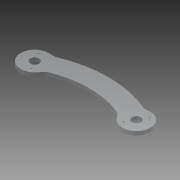
# Autodesk Inventor part: Femur
Saved by Autodesk Inventor 2015 (Build 190159000, 159)
## iProperties
Created: 2015-10-11
Part Number: Femur
Material: Generic
Document SubType Name: Modeling
Designer: styku
Density: 1 g/cm^3
Appearance: Clear - Blue
Mass: 4.92784 g
Surface Area: 41.7146 cm^2
Volume: 4.92784 cm^3
Author: styku
Autodesk Inventor part; units mm, degrees
ref_plane "YZ Plane" through (0, 0, 0) normal (1, 0, 0) x (0, 1, 0)
ref_plane "XZ Plane" through (0, 0, 0) normal (0, 1, 0) x (-1, 0, 0)
ref_plane "XY Plane" through (0, 0, 0) normal (0, 0, 1) x (1, 0, 0)
sketch "Sketch1" plane through (0, 0, 0) normal (0, 0, 1) x (1, 0, 0)
  line L0 (0, 107) -> (0, -103) construction
  line L1 (-117, 0) -> (116, 0) construction
  arc A0 (-38.3571, 10.8766) -> (-30.6918, -5.8614) centre (-40, 0) ccw
  arc A1 (30.6918, -5.8614) -> (38.3571, 10.8766) centre (40, 0) ccw
  arc A2 (40, 0) -> (-40, 0) centre (0, -69.282) ccw construction
  line L2 (-40, 13) -> (-40, -15) construction
  line L3 (40, 13) -> (40, -15) construction
  arc A3 (25.8036, -1.8505) -> (-25.8036, -1.8505) centre (0, -69.282) ccw
  arc A4 (33.0749, 11.5099) -> (-33.0749, 11.5099) centre (0, -69.282) ccw
  arc A5 (-38.3571, 10.8766) -> (-33.0749, 11.5099) centre (-36.8635, 20.7645) ccw
  arc A6 (-25.8036, -1.8505) -> (-30.6918, -5.8614) centre (-22.2297, -11.19) ccw
  arc A7 (33.0749, 11.5099) -> (38.3571, 10.8766) centre (36.8635, 20.7645) ccw
  arc A8 (30.6918, -5.8614) -> (25.8036, -1.8505) centre (22.2297, -11.19) ccw
  line L4 (-39.7655, 0.1354) -> (-60.5453, -11.8618) construction
  line L5 (-46.3958, 11.0778) -> (-33.6042, -11.0778) construction
  circle A9 centre (-43.75, 6.4952) radius 0.5
  circle A10 centre (-36.25, -6.4952) radius 0.5
  circle A11 centre (43.75, 6.4952) radius 0.5
  circle A12 centre (36.25, -6.4952) radius 0.5
  circle A13 centre (-40, 0) radius 3.5
  circle A14 centre (40, 0) radius 3.5
  point P0 (0, 0)
  dimension "d0" = 22
  dimension "d1" = 40
  dimension "d2" = 80
  dimension "d6" = 10
  dimension "d7" = 72.2
  dimension "d8" = 87.3
  dimension "d9" = 1
  dimension "d10" = 7.5
  dimension "d11" = 7
  constraints: 18 point on circle, 15 centre point, 12 end point, 9 tangent, 7 symmetric about line, 4 point on line, 3 equal radius, 2 concentric, 2 horizontal, 2 perpendicular, 2 vertical, 1 coincident, 1 midpoint, 5 other
  measures "d0" diameter of A0
  measures "d1" distance from line of L0 A0.centre
  measures "d2" radius of A2
  measures "d6" radius of A5
  measures "d7" radius of A3
  measures "d8" radius of A4
  measures "d9" diameter of A9
  measures "d10" distance from line of L4 A9.centre
  measures "d11" diameter of A13
extrude "Extrusion1" add sketch "Sketch1" along normal blind 3
body "Solid1"
